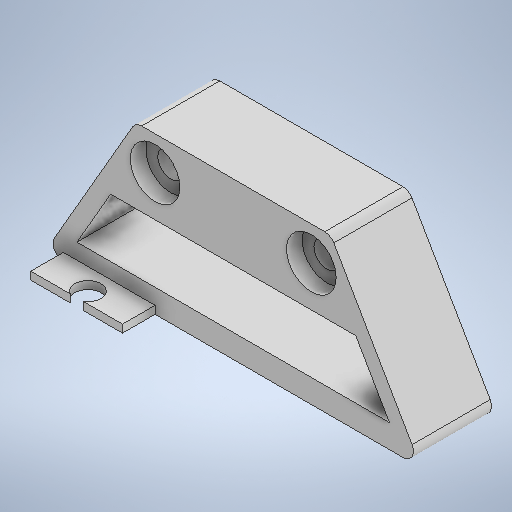
# Autodesk Inventor part: EngineMount - Big hole
Saved by Autodesk Inventor 2026.1 (Build 301233020, 233B)
## iProperties
Created: 2025-10-14
Part Number: EngineMount - Big hole
Material: Generic
Document SubType Name: Modeling
Designer: yo
Density: 1 g/cm^3
Appearance: Default
Author: yo
Autodesk Inventor part; units mm, degrees
ref_plane "YZ Plane" through (0, 0, 0) normal (1, 0, 0) x (0, 1, 0)
ref_plane "XZ Plane" through (0, 0, 0) normal (0, 1, 0) x (-1, 0, 0)
ref_plane "XY Plane" through (0, 0, 0) normal (0, 0, 1) x (1, 0, 0)
sketch "Sketch1" plane through (0, 0, 0) normal (0, 0, 1) x (1, 0, 0)
  line L0 (-65.2184, 0) -> (65.2184, 0)
  line L1 (-35.1673, 60.05) -> (35.1673, 60.05)
  circle A0 centre (-30, 47) radius 9.55
  line L2 (0, 60.05) -> (0, 0) construction
  circle A1 centre (-30, 47) radius 5
  circle A2 centre (30, 47) radius 9.55
  circle A3 centre (30, 47) radius 5
  arc A4 (-68.6825, 6) -> (-65.2184, 0) centre (-65.2184, 4) ccw
  arc A5 (-35.1673, 60.05) -> (-38.6314, 58.05) centre (-35.1673, 56.05) ccw
  line L3 (-68.6825, 6) -> (-38.6314, 58.05)
  arc A6 (65.2184, 0) -> (68.6825, 6) centre (65.2184, 4) ccw
  arc A7 (38.6314, 58.05) -> (35.1673, 60.05) centre (35.1673, 56.05) ccw
  line L4 (68.6825, 6) -> (38.6314, 58.05)
  line L5 (-65.2184, 3) -> (-30, 3)
  line L6 (-30, 3) -> (-30, 0)
  line L7 (-30, 0) -> (-65.2184, 0)
  line L8 (-65.2184, 0) -> (-65.2184, 3)
  line L9 (-30, 37.45) -> (0, 37.45) construction
  line L10 (-30, 3) -> (0, 3) construction
  line L11 (0, 37.45) -> (0, 3) construction
  line L12 (-60.0222, 9) -> (-47.0607, 31.45)
  line L13 (-47.0607, 31.45) -> (47.0607, 31.45)
  line L14 (47.0607, 31.45) -> (60.0222, 9)
  line L15 (60.0222, 9) -> (-60.0222, 9)
  point P0 (-65.2184, 1.5)
  point P1 (-47.6092, 0)
  point P2 (-65.2184, 0)
  point P3 (-30, 0)
  point P4 (-30, 1.5)
  point P5 (0, 20.225)
  point P6 (0, 20.225)
  point P7 (0, 20.225)
  dimension "d1" = 19.1
  dimension "d3" = 3.5
  dimension "d7" = 10
  dimension "d8" = 60
  dimension "d10" = 4
  dimension "d11" = 13
  dimension "d12" = 60
  dimension "d17" = 3
  dimension "d22" = 44
  dimension "d40" = 6
  dimension "d41" = 6
  dimension "d42" = 6
  dimension "d43" = 6
  constraints: 33 end point, 8 coincident, 8 point on circle, 7 centre point, 6 midpoint, 6 symmetric about line, 5 horizontal, 4 parallel, 4 tangent, 3 perpendicular, 3 vertical alignment, 2 point on line, 1 collinear, 1 equal radius, 1 horizontal alignment, 1 vertical, 6 other
  measures "d7" diameter of A1
  measures "d8" distance of A2.centre point (-30, 47)
  measures "d10" radius of A4
  measures "d11" distance from line of point (-30, 47) L3
  measures "d12" angle of L0 L3
  measures "d17" distance of L5.end L6.end
  measures "d22" distance from line of point (-30, 47) L5
  measures "d40" distance between parallel lines of L12 L3
  measures "d41" distance between parallel lines of L14 L4
  measures "d42" distance edge to line of A2 L13
  measures "d43" distance between parallel lines of L5 L15
extrude "Extrusion1" add sketch "Sketch1" along normal mid plane 30 contours L8 L5 L6 L0 | A4 L3 A5 L1 A7 L4 A6 L0 L6 L5 L8
extrude "Extrusion2" add sketch "Sketch1" along normal mid plane 18 contours A0 | A2
extrude "Extrusion3" add sketch "Sketch1" along normal blind 27.5 contours L8 L5 L6 L0
sketch "Sketch2" plane through (-65.2184, 3, 15) normal (0, 1, 0) x (1, 0, 0)
  line L0 (0, -12.5) -> (35.2184, -12.5) projected
  arc A0 (20.1092, -12.5) -> (15.1092, -12.5) centre (17.6092, -8.1699) ccw
  line L1 (35.2184, 0) -> (130.4367, 0) construction
  line L2 (35.2184, 0) -> (35.2184, -12.5) construction
  point P0 (65.2184, 15)
  point P1 (17.6092, -12.5)
  point P2 (17.6092, -3.1699)
  dimension "d21" = 5
  dimension "d25" = 5
  constraints: 3 point on circle, 2 point on line, 1 centre point, 1 midpoint, 1 vertical alignment
  measures "d21" radius of A0
  measures "d25" distance of A0.end A0.start
extrude "Extrusion4" cut sketch "Sketch2" against normal through all
body "Solid1"
